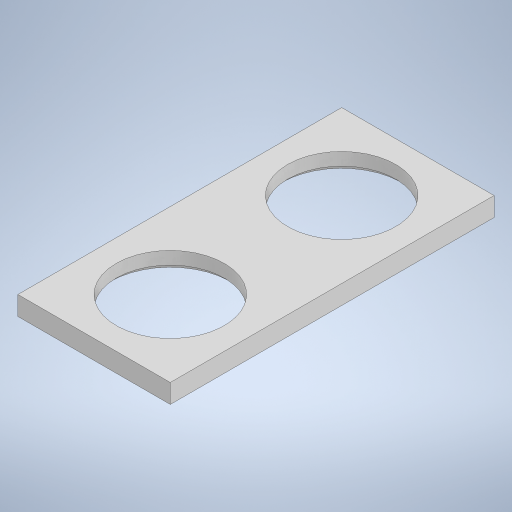
# Autodesk Inventor part: UltrasonicMountTest01
Saved by Autodesk Inventor 2024.2 (Build 282272000, 272)
## iProperties
Created: 2024-02-17
Part Number: UltrasonicMountTest01
Material: Generic
Document SubType Name: Modeling
Designer: ringl
Density: 1 g/cm^3
Appearance: Default
Author: ringl
Autodesk Inventor part; units mm, degrees
ref_plane "YZ Plane" through (0, 0, 0) normal (1, 0, 0) x (0, 1, 0)
ref_plane "XZ Plane" through (0, 0, 0) normal (0, 1, 0) x (-1, 0, 0)
ref_plane "XY Plane" through (0, 0, 0) normal (0, 0, 1) x (1, 0, 0)
sketch "Sketch1" plane through (0, 0, 0) normal (0, 1, 0) x (-1, 0, 0)
  circle A0 centre (0, 0) radius 8.5
  circle A1 centre (0, -27) radius 8.5
  line L0 (12, 12) -> (-12, 12)
  line L1 (-12, 12) -> (-12, -39)
  line L2 (-12, -39) -> (12, -39)
  line L3 (12, -39) -> (12, 12)
  point P0 (0, -39)
  dimension "d0" = 17
  dimension "d1" = 17
  dimension "d2" = 27
  dimension "d3" = 12
  dimension "d4" = 12
  dimension "d5" = 12
  dimension "d6" = 12
  constraints: 8 end point, 2 centre point, 2 parallel, 1 coincident, 1 horizontal, 1 midpoint, 1 perpendicular, 1 vertical alignment
  measures "d0" diameter of A0
  measures "d1" diameter of A1
  measures "d2" distance of point (0, 0) A1.centre
  measures "d3" distance from line of L0 point (0, 0)
  measures "d4" distance of point (0, -39) A1.centre
  measures "d5" distance from line of L1 point (0, 0)
  measures "d6" distance from line of L3 point (0, 0)
extrude "Extrusion1" add sketch "Sketch1" along normal blind 3
chamfer "Chamfer1" distance 1 angle 45 2 edges at (8.5, 0, 0) (8.5, 0, -27)
body "Solid1"
